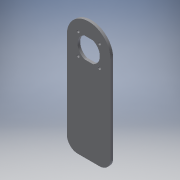
# Autodesk Inventor part: pG188Mount
Saved by Autodesk Inventor 2017 (Build 210142000, 142)
## iProperties
Created: 2017-02-20
Part Number: pG188Mount
Material: Generic
Document SubType Name: Sheet Metal
Designer: kingb
Density: 1 g/cm^3
Sheet Metal Rule: Default
Appearance: Default
Author: kingb
Autodesk Inventor part; units mm, degrees
ref_plane "YZ Plane" through (0, 0, 0) normal (1, 0, 0) x (0, 1, 0)
ref_plane "XZ Plane" through (0, 0, 0) normal (0, 1, 0) x (-1, 0, 0)
ref_plane "XY Plane" through (0, 0, 0) normal (0, 0, 1) x (1, 0, 0)
sketch "Sketch1" plane through (0, 0, 0) normal (0, 0, 1) x (1, 0, 0)
  line L0 (0, 0) -> (50.8, 0)
  line L1 (50.8, 0) -> (50.8, 139.7)
  line L2 (50.8, 139.7) -> (0, 139.7)
  line L3 (0, 139.7) -> (0, 0)
  dimension "d0" = 50.8
  dimension "d1" = 139.7
  measures "d0" distance of L2.end L1.end
  measures "d1" distance of L1.end L0.end
extrude "Plate1" add sketch "Sketch1" along normal blind 3.048
fillet "Corner Round1" radius 25.4 1 edges at (50.8, 139.7, 1.524)
fillet "Corner Round1" radius 25.4 1 edges at (0, 139.7, 1.524)
fillet "Corner Round2" radius 12.7 2 edges at (50.8, 0, 1.524) (0, 0, 1.524)
sketch "Sketch2" plane through (0, 0, 0) normal (0, 0, -1) x (-1, 0, 0)
  arc A0 (-20.4, 99.125) -> (-20.4, 123.125) centre (-25.4, 111.125) ccw projected
  line L0 (-20.4, 123.125) -> (-30.4, 123.125) projected
  line L1 (-30.4, 99.125) -> (-20.4, 99.125) projected
  arc A1 (-30.4, 123.125) -> (-30.4, 99.125) centre (-25.4, 111.125) ccw projected
  circle A2 centre (-13.0256, 98.7506) radius 1.65 projected
  circle A3 centre (-37.7744, 123.4994) radius 1.65 projected
  circle A4 centre (-13.0256, 123.4994) radius 1.65 projected
  circle A5 centre (-37.7744, 98.7506) radius 1.65 projected
  point P0 (0, 0)
extrude "Extrusion1" cut sketch "Sketch2" against normal up to surface (3.048 mm away)
sketch "Sketch3" plane through (0, 0, 3.048) normal (0, 0, 1) x (1, 0, 0)
  circle A0 centre (12.7, 76.2) radius 2.9337 projected
  circle A1 centre (38.1, 76.2) radius 2.9337 projected
  circle A2 centre (38.1, 44.45) radius 2.9337 projected
  circle A3 centre (12.7, 44.45) radius 2.9337 projected
  circle A4 centre (12.7, 12.7) radius 2.9337 projected
  circle A5 centre (38.1, 12.7) radius 2.9337 projected
  circle A6 centre (12.7, 12.7) radius 2.9337 projected
  point P0 (0, 0)
extrude "Extrusion2" cut sketch "Sketch3" against normal up to surface (3.048 mm away)
equation "\"BendRadius\" = Thickness"
equation "\"BendReliefWidth\" = Thickness"
equation "\"BendReliefDepth\" = 0.5 * Thickness"
equation "\"CornerReliefSize\" = 4 * Thickness"
equation "\"MinimumRemnant\" = 2 * Thickness"
equation "\"TransitionRadius\" = BendRadius"
equation "\"JacobiRadiusSize\" = Thickness"
equation "\"GapSize\" = Thickness"
equation "\"d2\" = BendRadius"
equation "\"Thickness\" = 3.048"
body "Solid1"
